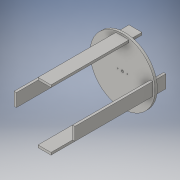
# Autodesk Inventor part: Zoetrope_Board
Saved by Autodesk Inventor 2016 (Build 200138000, 138)
## iProperties
Created: 2019-01-15
Part Number: Zoetrope_Board
Material: Generic
Document SubType Name: Modeling
Designer: student
Density: 1 g/cm^3
Appearance: Default
Author: student
Autodesk Inventor part; units mm, degrees
ref_plane "YZ Plane" through (0, 0, 0) normal (1, 0, 0) x (0, 1, 0)
ref_plane "XZ Plane" through (0, 0, 0) normal (0, 1, 0) x (-1, 0, 0)
ref_plane "XY Plane" through (0, 0, 0) normal (0, 0, 1) x (1, 0, 0)
sketch "Sketch1" plane through (0, 0, 0) normal (0, 0, 1) x (1, 0, 0)
  circle A0 centre (0, 0) radius 63.5
  line L0 (0, 0) -> (9.525, 0) construction
  line L1 (0, 0) -> (-9.525, 0) construction
  circle A1 centre (-9.525, 0) radius 0.9525
  circle A2 centre (9.525, 0) radius 0.9525
  circle A3 centre (0, 0) radius 2.2225
  dimension "d0" = 127
  dimension "d2" = 9.525
  dimension "d3" = 9.525
  dimension "d4" = 1.905
  dimension "d5" = 1.905
  dimension "d6" = 4.445
  constraints: 5 coincident, 4 centre point, 4 end point, 2 horizontal
  measures "d0" diameter of A0
  measures "d2" distance of L0.start L0.end
  measures "d3" distance of L0.start L1.end
  measures "d4" diameter of A1
  measures "d5" diameter of A2
  measures "d6" diameter of A3
extrude "Extrusion1" add sketch "Sketch1" along normal blind 4.572
sketch "Sketch2" plane through (0, 0, 4.572) normal (0, 0, 1) x (1, 0, 0)
  circle A0 centre (0, 0) radius 2.2225 projected
  line L0 (0, 0) -> (57.15, 0)
  line L1 (0, 0) -> (0, -57.15)
  line L2 (0, 0) -> (-57.15, 0)
  line L3 (0, 0) -> (57.15, 0) construction
  line L4 (0, 0) -> (0, 57.15)
  line L5 (-54.864, -12.7) -> (-59.436, -12.7)
  line L6 (-59.436, -12.7) -> (-59.436, 12.7)
  line L7 (-59.436, 12.7) -> (-54.864, 12.7)
  line L8 (-54.864, 12.7) -> (-54.864, -12.7)
  line L9 (-54.864, -12.7) -> (-59.436, 12.7) construction
  line L10 (-59.436, -12.7) -> (-54.864, 12.7) construction
  line L11 (-12.7, 54.864) -> (12.7, 54.864)
  line L12 (12.7, 54.864) -> (12.7, 59.436)
  line L13 (12.7, 59.436) -> (-12.7, 59.436)
  line L14 (-12.7, 59.436) -> (-12.7, 54.864)
  line L15 (-12.7, 54.864) -> (12.7, 59.436) construction
  line L16 (12.7, 54.864) -> (-12.7, 59.436) construction
  line L17 (59.436, -12.7) -> (54.864, -12.7)
  line L18 (54.864, -12.7) -> (54.864, 12.7)
  line L19 (54.864, 12.7) -> (59.436, 12.7)
  line L20 (59.436, 12.7) -> (59.436, -12.7)
  line L21 (59.436, -12.7) -> (54.864, 12.7) construction
  line L22 (54.864, -12.7) -> (59.436, 12.7) construction
  line L23 (-12.7, -59.436) -> (12.7, -59.436)
  line L24 (12.7, -59.436) -> (12.7, -54.864)
  line L25 (12.7, -54.864) -> (-12.7, -54.864)
  line L26 (-12.7, -54.864) -> (-12.7, -59.436)
  line L27 (-12.7, -59.436) -> (12.7, -54.864) construction
  line L28 (12.7, -59.436) -> (-12.7, -54.864) construction
  dimension "d10" = 57.15
  dimension "d11" = 57.15
  dimension "d12" = 57.15
  dimension "d13" = 180
  dimension "d14" = 57.15
  dimension "d15" = 4.572
  dimension "d16" = 25.4
  dimension "d17" = 25.4
  dimension "d18" = 4.572
  dimension "d19" = 4.572
  dimension "d20" = 25.4
  dimension "d21" = 4.572
  constraints: 58 end point, 8 midpoint, 8 parallel, 7 horizontal, 4 perpendicular, 2 vertical, 1 collinear
  measures "d10" distance of L0.start L0.end
  measures "d11" distance of L0.start L1.end
  measures "d12" distance of L0.start L2.end
  measures "d13" angle of L2 L3
  measures "d14" distance of L0.start L4.end
  measures "d15" distance of L6.end L7.end
  measures "d16" distance of L5.end L6.end
  measures "d17" distance of L13.end L12.end
  measures "d18" distance of L12.end L11.end
  measures "d19" distance of L18.end L19.end
  measures "d20" distance of L17.end L18.end
  measures "d21" distance of L24.end L23.end
extrude "Extrusion2" add sketch "Sketch2" along normal blind 152.4 and the other way blind 25.4 contours L5 L6 L7 L8 | L14 L13 L12 L11 | L17 L18 L19 L20 | L26 L25 L24 L23
body "Solid1"
